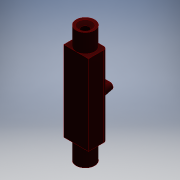
# Autodesk Inventor part: tracks_center
Saved by Autodesk Inventor 2016 (Build 200138000, 138)
## iProperties
Created: 2016-05-02
Part Number: tracks_center
Material: ABS Plastic
Document SubType Name: Modeling
Designer: Henrik Samuelsson
Density: 1.06 g/cm^3
Appearance: Smooth - White
Author: Henrik Samuelsson
Autodesk Inventor part; units mm, degrees
ref_plane "YZ Plane" through (0, 0, 0) normal (1, 0, 0) x (0, 1, 0)
ref_plane "XZ Plane" through (0, 0, 0) normal (0, 1, 0) x (-1, 0, 0)
sketch "Sketch1" plane through (0, 0, 0) normal (0, 1, 0) x (-1, 0, 0)
  line L0 (0, 0) -> (8, 0)
  line L1 (8, 0) -> (8, -26)
  line L2 (8, -26) -> (0, -26)
  line L3 (0, -26) -> (0, 0)
  dimension "d0" = 8
  dimension "d1" = 26
  constraints: 8 end point, 2 parallel, 1 horizontal, 1 perpendicular
  measures "d0" distance of L1.end L2.end
  measures "d1" distance of L1.end L0.end
extrude "Extrusion1" add sketch "Sketch1" along normal blind 6
sketch "Sketch2" plane through (-8, 0, 0) normal (0, 0, 1) x (1, 0, 0)
  circle A0 centre (4, 3) radius 3
  line L0 (8, 0) -> (0, 0) projected
  line L1 (0, 0) -> (0, 6) projected
  dimension "d4" = 6
  dimension "d5" = 3
  dimension "d6" = 4
  constraints: 1 centre point
  measures "d4" diameter of A0
  measures "d5" distance from line of L0 A0.centre
  measures "d6" distance from line of L1 A0.centre
extrude "Extrusion2" add sketch "Sketch2" along normal blind 6
sketch "Sketch3" plane through (0, 0, -26) normal (0, 0, -1) x (-1, 0, 0)
  arc A0 (4, 0) -> (4, 6) centre (4, 3) ccw projected
  arc A1 (4, 6) -> (4, 0) centre (4, 3) ccw projected
  circle A2 centre (4, 3) radius 3
  point P0 (0, 0)
  constraints: 1 coincident, 1 vertical alignment, 2 other
extrude "Extrusion3" add sketch "Sketch3" along normal blind 6
ref_plane "Work Plane1" through (0, 9, 0) normal (0, 1, 0) x (1, 0, 0)
sketch "Sketch7" plane through (0, 6, 0) normal (0, 1, 0) x (1, 0, 0)
  line L0 (-2, 13) -> (-6, 13) construction
  line L1 (-4.5266, -6) -> (-4.5266, 32) projected
  line L2 (-2, 14.5) -> (-6, 14.5)
  line L3 (-6, 11.5) -> (-2, 11.5)
  arc A0 (-2, 11.5) -> (-2, 14.5) centre (-2, 13) ccw
  arc A1 (-6, 14.5) -> (-6, 11.5) centre (-6, 13) ccw
  line L4 (-8, 26) -> (-8, 0) projected
  line L5 (-4, 0) -> (0, 0) projected
  point P0 (-4, 13)
  dimension "d26" = 3
  dimension "d27" = 4
  dimension "d28" = 4
  dimension "d29" = 13
  constraints: 8 end point, 4 point on circle, 4 tangent, 2 centre point, 1 midpoint, 1 parallel, 1 perpendicular
  measures "d26" diameter of A1
  measures "d27" distance from line of L4 point (-4, 13)
  measures "d28" distance of L0.end L0.start
  measures "d29" distance from line of L5 point (-4, 13)
sketch "Sketch8" plane through (0, 9, 0) normal (0, 1, 0) x (1, 0, 0)
  line L0 (-2, 13) -> (-6, 13) construction
  line L1 (-2, 14) -> (-6, 14)
  line L2 (-6, 12) -> (-2, 12)
  arc A0 (-2, 12) -> (-2, 14) centre (-2, 13) ccw
  arc A1 (-6, 14) -> (-6, 12) centre (-6, 13) ccw
  line L3 (-4, 13) -> (0, 13) construction
  line L4 (-8, 26) -> (-8, 0) projected
  line L5 (-4, 0) -> (0, 0) projected
  dimension "d30" = 2
  dimension "d31" = 180
  dimension "d32" = 2
  dimension "d33" = 4
  dimension "d34" = 13
  constraints: 10 end point, 4 point on circle, 4 tangent, 2 centre point, 2 horizontal, 1 collinear, 1 midpoint, 1 parallel
  measures "d30" distance of L3.start L0.end
  measures "d31" angle of L0 L3
  measures "d32" diameter of A1
  measures "d33" distance from line of L4 L3.start
  measures "d34" distance from line of L5 L3.start
loft "Loft1" add profiles "Sketch7", "Sketch8"
hole "Hole2" at (-3.899, 2.8555, -32) direction (0, 0, 1) diameter 2.5 end through all
chamfer "Chamfer1" distance 1 angle 45 1 edges at (-3.899, 1.6055, 6)
chamfer "Chamfer2" distance 1 angle 45 1 edges at (-3.899, 1.6055, -32)
fillet "Fillet1" radius 1 2 edges at (-8, 6, -13) (0, 6, -13)
body "Solid1"
